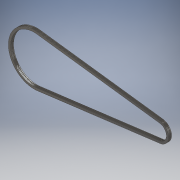
# Autodesk Inventor part: IntakeChain
Saved by Autodesk Inventor 2018.3 (Build 223284000, 284)
## iProperties
Created: 2020-02-08
Part Number: IntakeChain
Material: Steel
Document SubType Name: Modeling
Designer: Myers
Mass: 162.099 g
Surface Area: 176.571 cm^2
Volume: 20.6495 cm^3
Density: 7.85 g/cm^3
Appearance: Diamond Plate
Author: Myers
Autodesk Inventor part; units mm, degrees
ref_plane "YZ Plane" through (0, 0, 0) normal (1, 0, 0) x (0, 1, 0)
ref_plane "XZ Plane" through (0, 0, 0) normal (0, 1, 0) x (-1, 0, 0)
ref_plane "XY Plane" through (0, 0, 0) normal (0, 0, 1) x (1, 0, 0)
sketch "Sketch2" plane through (0, 0, 0) normal (0, 0, 1) x (1, 0, 0)
  arc A0 (2.7403, -21.4154) -> (2.7403, 21.4154) centre (0, 0) ccw
  arc A1 (-322.1404, 62.9864) -> (-322.1404, -62.9864) centre (-330.2, 0) ccw
  line L0 (-322.1404, 62.9864) -> (2.7403, 21.4154)
  line L1 (2.7403, -21.4154) -> (-322.1404, -62.9864)
  dimension "d1" = 330.2
  dimension "d3" = 43.18
  dimension "d4" = 127
  constraints: 4 end point, 4 point on circle, 4 tangent, 2 centre point, 1 coincident, 1 horizontal alignment
  measures "d1" distance of A0.centre A1.centre
  measures "d3" diameter of A0
  measures "d4" diameter of A1
sketch "Sketch3" plane through (0, 0, 0) normal (0, 1, 0) x (-1, 0, 0)
  line L0 (-2.7403, 0) -> (-21.59, 0) projected
  line L1 (-26.1366, 3.9497) -> (-20.3454, 3.9497)
  line L2 (-20.3454, 3.9497) -> (-20.3454, 1.5875)
  line L3 (-20.3454, 1.5875) -> (-21.59, 1.5875)
  line L4 (-21.59, 1.5875) -> (-21.59, -1.5875)
  line L5 (-21.59, -1.5875) -> (-20.3454, -1.5875)
  line L6 (-20.3454, -1.5875) -> (-20.3454, -3.9497)
  line L7 (-20.3454, -3.9497) -> (-26.1366, -3.9497)
  line L8 (-26.1366, -3.9497) -> (-26.1366, -1.5875)
  line L9 (-26.1366, -1.5875) -> (-24.892, -1.5875)
  line L10 (-24.892, -1.5875) -> (-24.892, 1.5875)
  line L11 (-24.892, 1.5875) -> (-26.1366, 1.5875)
  line L12 (-26.1366, 3.9497) -> (-26.1366, 1.5875)
  point P0 (0, 0)
  point P1 (-24.892, 0)
  dimension "d8" = 5.7912
  dimension "d9" = 7.8994
  dimension "d10" = 3.175
  dimension "d11" = 3.302
  constraints: 24 end point, 8 perpendicular, 8 point on line, 2 collinear, 2 midpoint, 1 horizontal, 1 horizontal alignment
  measures "d8" distance of L6.end L7.end
  measures "d9" distance between parallel lines of L7 L1
  measures "d10" distance of L9.end L10.end
  measures "d11" distance between parallel lines of L10 L4
sweep "Sweep1" add profiles "Sketch3" path "Sketch2"
body "Solid2"
